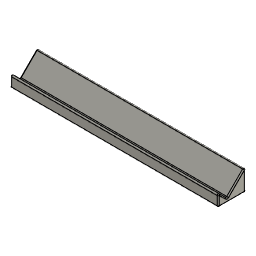
qwirkle-stand (Autodesk Fusion 360 design; units mm, degrees)
Autodesk Fusion 360 part; units mm, degrees
sketch "Skizze1" plane through (0, 0, 0) normal (1, 0, 0) x (0, 1, 0)
  line L0 (0, 0.9738) -> (0, 9.5858)
  line L1 (1.7071, 10.2929) -> (7.7782, 4.2218)
  line L2 (0, 12) -> (12, 12) construction
  line L3 (9.1924, 4.2218) -> (24.4558, 19.4853)
  line L4 (8.4853, 3.5147) -> (33.4853, 3.5147) construction
  line L5 (26.163, 18.7782) -> (26.163, 0.9804)
  line L6 (25.1897, 0.0069) -> (0.9738, 0.0003)
  arc A0 (1.7071, 10.2929) -> (0, 9.5858) centre (1, 9.5858) ccw
  arc A1 (26.163, 18.7782) -> (24.4558, 19.4853) centre (25.163, 18.7782) ccw
  arc A2 (0, 0.9738) -> (0.9738, 0.0003) centre (0.9735, 0.9738) ccw
  arc A3 (25.1897, 0.0069) -> (26.163, 0.9804) centre (25.1894, 0.9804) ccw
  arc A4 (7.7782, 4.2218) -> (9.1924, 4.2218) centre (8.4853, 4.9289) ccw
  point P0 (26.163, 21.1924)
  dimension "d1" = 12
  dimension "d2" = 12
  dimension "d3" = 45
  dimension "d4" = 45
  dimension "d5" = 25
  dimension "d6" = 1
  dimension "d7" = 0.9735
  dimension "d10" = 1
  constraint vertical L0
  constraint horizontal L2
  constraint horizontal L4
  constraint perpendicular L4 L5
  constraint coincident L2.start L0
  constraint coincident L2.start L1
  constraint tangent L0 A0
  constraint tangent L1 A0
  constraint coincident P0 L3
  constraint coincident P0 L5
  constraint tangent L3 A1
  constraint tangent L5 A1
  constraint equal A0 A1
  constraint coincident origin L0
  constraint tangent L0 A2
  constraint tangent L6 A2
  constraint tangent L5 A3
  constraint tangent L6 A3
  constraint equal A2 A3
  constraint coincident L4.start L1
  constraint coincident L4.start L3
  constraint tangent L1 A4
  constraint tangent L3 A4
  measures "d1" distance of origin L2.start
  measures "d2" distance of L2.start L4.start
  measures "d3" angle of L1 L2
  measures "d4" angle of L3 L4
  measures "d5" distance of L4.start P0
  measures "d6" radius of A0
  measures "d7" radius of A2
  measures "d10" radius of A4
extrude "Extrusion1" add sketch "Skizze1" along normal blind 200
fillet "Abrundung1" radius 1 10 edges at (200, 13.0817, 0.0036) (200, 25.8779, 0.2922) (200, 26.163, 9.8793) (200, 25.5456, 19.7021) (200, 16.8241, 11.8536) (200, 8.4853, 3.9289) (200, 4.7426, 7.2574) (200, 0.6173, 10.5097) (200, 0, 5.2798) (200, 0.2852, 0.2853)
fillet "Abrundung1" radius 1 10 edges at (0, 0.6173, 10.5097) (0, 4.7426, 7.2574) (0, 8.4853, 3.9289) (0, 16.8241, 11.8536) (0, 25.5456, 19.7021) (0, 26.163, 9.8793) (0, 25.8779, 0.2922) (0, 13.0817, 0.0036) (0, 0.2852, 0.2853) (0, 0, 5.2798)
